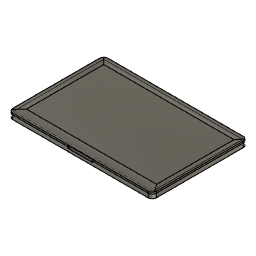
E-Ink Frame (v1) (Autodesk Fusion 360 design; units mm, degrees)
Autodesk Fusion 360 part; units mm, degrees
note: some values were not read from the file. Chosen so that the rebuilt part matches the saved one: which pieces of a blend or face edit are solid.
sketch "Sketch1" plane through (0, 0, 0) normal (0, 0, 1) x (1, 0, 0)
  line L0 (0, 0) -> (176, 0)
  line L1 (176, 0) -> (176, 116.5)
  line L2 (176, 116.5) -> (0, 116.5)
  line L3 (0, 116.5) -> (0, 0)
  dimension "d1" = 176
  dimension "d2" = 116.5
  constraint horizontal L0
  constraint vertical L1
  constraint horizontal L2
  constraint vertical L3
  constraint coincident L0.start L3.end
  measures "d1" distance of L0.start L0.end
  measures "d2" distance of L0.start L2.end
extrude "Extrude1" add sketch "Sketch1" along normal blind 4 makes body 1
sketch "Sketch3" plane through (0, 0, 4) normal (0, 0, 1) x (-1, 0, 0)
  line L0 (0, -116.5) -> (0, 0)
  line L1 (0, 0) -> (-176, 0)
  line L2 (-176, 0) -> (-176, -116.5)
  line L3 (-176, -116.5) -> (0, -116.5)
  line L4 (-3, -3) -> (-173, -3)
  line L5 (-173, -3) -> (-173, -113.5)
  line L6 (-173, -113.5) -> (-3, -113.5)
  line L7 (-3, -113.5) -> (-3, -3)
  line L8 (-8.2, -13.5) -> (-167.8, -13.5)
  line L9 (-167.8, -13.5) -> (-167.8, -108.3)
  line L10 (-167.8, -108.3) -> (-8.2, -108.3)
  line L11 (-8.2, -108.3) -> (-8.2, -13.5)
  dimension "d7" = 170
  dimension "d8" = 110.5
  constraint horizontal L4
  constraint vertical L5
  constraint horizontal L6
  constraint vertical L7
  constraint horizontal L8
  constraint vertical L9
  constraint horizontal L10
  constraint vertical L11
  measures "d7" distance of L4.start L4.end
  measures "d8" distance of L4.start L6.end
extrude "Extrude2" add sketch "Sketch3" along normal blind 3 contours L0 L1 L2 L3 | L4 L5 L6 L7 bodies 1
sketch "Gap cut for screen" plane through (0, 0, 0) normal (0, -1, 0) x (1, 0, 0)
  line L0 (0, 0) -> (176, 0)
  line L1 (176, 0) -> (176, 7)
  line L2 (176, 7) -> (0, 7)
  line L3 (0, 7) -> (0, 0)
  line L4 (0, 0) -> (3, 0)
  line L5 (3, 0) -> (3, 5)
  line L6 (0, 5) -> (0, 0)
  line L7 (0, 6) -> (0, 5)
  line L8 (173, 6) -> (173, 5)
  line L9 (3, 5) -> (0, 5)
  line L10 (0, 5) -> (0, 6)
  line L11 (3, 6) -> (3, 5)
  line L12 (3, 5) -> (173, 5)
  line L13 (173, 5) -> (173, 6)
  line L14 (173, 6) -> (3, 6)
  dimension "d15" = 3
  dimension "d16" = 5
  dimension "d17" = 1
  constraint horizontal L4
  constraint vertical L5
  constraint vertical L6
  constraint coincident L0.start L3.end
  constraint vertical L7
  constraint vertical L8
  constraint horizontal L9
  constraint vertical L10
  constraint vertical L11
  constraint horizontal L12
  constraint vertical L13
  constraint horizontal L14
  measures "d15" distance of L0.start L4.end
  measures "d16" distance of L0.start L6.start
  measures "d17" distance of L6.start L7.start
extrude "Extrude3" cut sketch "Gap cut for screen" against normal up to surface (110.5 mm away) from surface at -3 contours L8 L11 L12 L13 L14 bodies 1
extrude "Extrude4" add sketch "Sketch3" along normal blind 1 contours L8 L9 L10 L11 bodies 1
sketch "Sketch5" plane through (0, 0, 0) normal (0, -1, 0) x (1, 0, 0)
  line L0 (0, 0) -> (176, 0)
  line L1 (176, 0) -> (176, 7)
  line L2 (176, 7) -> (0, 7)
  line L3 (0, 7) -> (0, 0)
  line L4 (0, 0) -> (74, 0)
  line L5 (74, 0) -> (102, 0)
  line L6 (102, 0) -> (176, 0)
  line L7 (102, 0) -> (176, 0)
  line L8 (102, 5) -> (74, 5)
  line L9 (74, 6) -> (74, 5)
  line L10 (74, 6) -> (102, 6)
  line L11 (102, 6) -> (102, 5)
  dimension "d24" = 74
  dimension "d25" = 28
  dimension "d26" = 74
  dimension "d27" = 5
  dimension "d28" = 28
  dimension "d29" = 1
  constraint coincident L0.start L3.end
  constraint perpendicular L3 L4
  constraint parallel L0 L5
  constraint coincident L0.end L1.start
  constraint parallel L6 L7
  constraint vertical L9
  constraint perpendicular L8 L11
  measures "d24" distance of L0.start L4.end
  measures "d25" distance of L4.end L5.end
  measures "d26" distance of L5.end L0.end
  measures "d27" distance of L5.end L8.start
  measures "d28" distance of L8.start L8.end
  measures "d29" distance of L8.end L9.start
extrude "Extrude5" cut sketch "Sketch5" against normal blind 3 contours L8 L9 L10 L11 bodies 1
fillet "Fillet1" radius 110 4 edges at (8.2, 60.9, 7) (88, 108.3, 7) (88, 13.5, 7) (167.8, 60.9, 7) on bodies 1
fillet "Fillet2" radius 1.5 4 edges at (88, 0, 6) (74, 0, 5.5) (88, 0, 5) (102, 0, 5.5) on bodies 1
fillet "Fillet3" radius 5 4 edges at (176, 116.5, 3.5) (0, 116.5, 3.5) (176, 0, 3.5) (0, 0, 3.5) on bodies 1
ref_plane "WorkPlane2" through (88, 57.5, 5) normal (0, 0, 1) x (1, 0, 0)
split "Split1" by plane through (88, 57.5, 5) normal (0, 0, 1) bodies 1 makes body 2 at (83.3333, 10, 6)
named bodies: "BottomFrame", "TopFrame"
